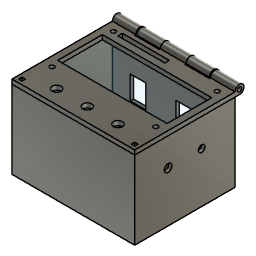
My_STM32_Box v11 (Autodesk Fusion 360 design; units mm, degrees)
Autodesk Fusion 360 part; units mm, degrees
note: some values were not read from the file. Set by a fixed rule: which sketch regions a step uses.
sketch "Sketch1" plane through (0, 0, 0) normal (0, 0, 1) x (1, 0, 0)
  line L0 (0, 0) -> (110, 0)
  line L1 (110, 0) -> (110, 70)
  line L2 (110, 70) -> (0, 70)
  line L3 (0, 70) -> (0, 0)
  dimension "d1" = 110
  dimension "d2" = 70
  constraint horizontal L0
  constraint vertical L1
  constraint horizontal L2
  constraint vertical L3
  constraint coincident L0.start L3.end
  measures "d1" distance of L0.start L0.end
  measures "d2" distance of L0.start L2.end
sketch "Sketch2" plane through (0, 0, 3) normal (0, 0, 1) x (-1, 0, 0)
  line L0 (0, -70) -> (0, 0)
  line L1 (0, 0) -> (-110, 0)
  line L2 (-110, 0) -> (-110, -70)
  line L3 (-110, -70) -> (0, -70)
  line L4 (-5, -14) -> (-105, -14)
  line L5 (-105, -14) -> (-105, -56)
  line L6 (-105, -56) -> (-5, -56)
  line L7 (-5, -56) -> (-5, -14)
  dimension "d10" = 100
  dimension "d11" = 42
  constraint horizontal L4
  constraint vertical L5
  constraint horizontal L6
  constraint vertical L7
  measures "d10" distance of L4.start L4.end
  measures "d11" distance of L4.start L6.end
sketch "Sketch3" plane through (0, 0, 3) normal (0, 0, 1) x (-1, 0, 0)
  line L0 (-105, -14) -> (-5, -14)
  line L1 (-5, -14) -> (-5, -56)
  line L2 (-5, -56) -> (-105, -56)
  line L3 (-105, -56) -> (-105, -14)
  line L4 (0, -70) -> (0, 0)
  line L5 (0, 0) -> (-110, 0)
  line L6 (-110, 0) -> (-110, -70)
  line L7 (-110, -70) -> (0, -70)
  line L8 (-12, -63) -> (-55, -63)
  line L9 (-55, -63) -> (-55, -65)
  line L10 (-55, -65) -> (-12, -65)
  line L11 (-12, -65) -> (-12, -63)
  dimension "d14" = 43
  dimension "d15" = 2
  constraint horizontal L8
  constraint vertical L9
  constraint horizontal L10
  constraint vertical L11
  measures "d14" distance of L8.start L8.end
  measures "d15" distance of L8.start L10.end
sketch "Sketch4" plane through (0, 0, 3) normal (0, 0, 1) x (-1, 0, 0)
  line L0 (-55, -63) -> (-12, -63)
  line L1 (-12, -63) -> (-12, -65)
  line L2 (-12, -65) -> (-55, -65)
  line L3 (-55, -65) -> (-55, -63)
  line L4 (-105, -14) -> (-5, -14)
  line L5 (-5, -14) -> (-5, -56)
  line L6 (-5, -56) -> (-105, -56)
  line L7 (-105, -56) -> (-105, -14)
  line L8 (0, -70) -> (0, 0)
  line L9 (0, 0) -> (-110, 0)
  line L10 (-110, 0) -> (-110, -70)
  line L11 (-110, -70) -> (0, -70)
  circle A0 centre (-7.3, -7.3) radius 2
  dimension "d18" = 4
  measures "d18" diameter of A0
sketch "Sketch5" plane through (0, 0, 3) normal (0, 0, 1) x (-1, 0, 0)
  circle A0 centre (-7.3, -7.3) radius 2
  line L0 (-55, -63) -> (-12, -63)
  line L1 (-12, -63) -> (-12, -65)
  line L2 (-12, -65) -> (-55, -65)
  line L3 (-55, -65) -> (-55, -63)
  line L4 (-105, -14) -> (-5, -14)
  line L5 (-5, -14) -> (-5, -56)
  line L6 (-5, -56) -> (-105, -56)
  line L7 (-105, -56) -> (-105, -14)
  line L8 (0, -70) -> (0, 0)
  line L9 (0, 0) -> (-110, 0)
  line L10 (-110, 0) -> (-110, -70)
  line L11 (-110, -70) -> (0, -70)
  circle A1 centre (-102.7, -7.3) radius 2
  dimension "d21" = 4
  measures "d21" diameter of A1
sketch "Sketch6" plane through (0, 0, 3) normal (0, 0, 1) x (-1, 0, 0)
sketch "Sketch7" plane through (0, 0, 0) normal (0, 0, 1) x (1, 0, 0)
  line L0 (0, 0) -> (110, 0)
  line L1 (110, 0) -> (110, 70)
  line L2 (110, 70) -> (0, 70)
  line L3 (0, 70) -> (0, 0)
  dimension "d24" = 110
  dimension "d25" = 70
  constraint horizontal L0
  constraint vertical L1
  constraint horizontal L2
  constraint vertical L3
  constraint coincident L0.start L3.end
  measures "d24" distance of L0.start L0.end
  measures "d25" distance of L0.start L2.end
extrude "Extrude7" add sketch "Sketch7" along normal blind 4 makes body 1
sketch "Sketch8" plane through (0, 0, 4) normal (0, 0, 1) x (-1, 0, 0)
  line L0 (0, -70) -> (0, 0)
  line L1 (0, 0) -> (-110, 0)
  line L2 (-110, 0) -> (-110, -70)
  line L3 (-110, -70) -> (0, -70)
  line L4 (0, 0) -> (-8.5, 0)
  line L5 (-8.5, 0) -> (-8.5, -7.5)
  line L6 (-8.5, -7.5) -> (-101.5, -7.5)
  line L7 (-101.5, -62.5) -> (-8.5, -62.5)
  circle A0 centre (-8.5, -62.5) radius 2
  circle A1 centre (-101.5, -62.5) radius 2
  circle A2 centre (-8.5, -7.5) radius 2
  circle A3 centre (-101.5, -7.5) radius 2
  line L8 (0, 0) -> (-4, 0)
  line L9 (-4, 0) -> (-4, -13)
  line L10 (-4, -13) -> (0, -13)
  line L11 (0, -13) -> (0, 0)
  line L12 (-4, -13) -> (-106, -13)
  line L13 (-106, -13) -> (-106, -57)
  line L14 (-106, -57) -> (-4, -57)
  line L15 (-4, -57) -> (-4, -13)
  line L16 (-14, -61) -> (-56, -61)
  line L17 (-56, -61) -> (-56, -65)
  line L18 (-56, -65) -> (-14, -65)
  line L19 (-14, -65) -> (-14, -61)
  dimension "d28" = 8.5
  dimension "d29" = 7.5
  dimension "d30" = 93
  dimension "d31" = 55
  dimension "d32" = 4
  dimension "d33" = 4
  dimension "d34" = 4
  dimension "d35" = 4
  dimension "d36" = 4
  dimension "d37" = 13
  dimension "d38" = 102
  dimension "d39" = 44
  dimension "d40" = 42
  constraint coincident L0.end L1.start
  constraint perpendicular L0 L4
  constraint perpendicular L4 L5
  constraint horizontal L6
  constraint horizontal L7
  constraint coincident L7.end A0.centre
  constraint coincident L7.start A1.centre
  constraint coincident L5.end L6.start
  constraint coincident L6.end A3.centre
  constraint horizontal L8
  constraint vertical L9
  constraint horizontal L10
  constraint vertical L11
  constraint horizontal L12
  constraint vertical L13
  constraint horizontal L14
  constraint vertical L15
  constraint horizontal L16
  constraint vertical L17
  constraint horizontal L18
  constraint vertical L19
  measures "d28" distance of L0.end L4.end
  measures "d29" distance of L4.end L5.end
  measures "d30" distance of L5.end L6.end
  measures "d31" distance of L5.end L7.end
  measures "d32" diameter of A0
  measures "d33" diameter of A1
  measures "d34" diameter of A2
  measures "d35" diameter of A3
  measures "d36" distance of L0.end L8.end
  measures "d37" distance of L0.end L10.end
  measures "d38" distance of L9.end L12.end
  measures "d39" distance of L9.end L14.end
  measures "d40" distance of L16.start L16.end
extrude "Extrude8" cut sketch "Sketch8" against normal blind 4 contours L12 L13 L14 L15 | L5 L6 A2 | L5 L6 A2 | L7 L16 L17 L19 | L7 L17 L18 L19 | A0 | A1 | A3 bodies 1
sketch "Sketch9" plane through (110, 0, 0) normal (1, 0, 0) x (0, 1, 0)
  line L0 (0, 0) -> (70, 0)
  line L1 (70, 0) -> (70, 4)
  line L2 (70, 4) -> (0, 4)
  line L3 (0, 4) -> (0, 0)
sketch "Sketch10" plane through (110, 0, 0) normal (1, 0, 0) x (0, 1, 0)
sketch "Sketch11" plane through (0, 0, 0) normal (-1, 0, 0) x (0, -1, 0)
  line L0 (-70, 0) -> (0, 0)
  line L1 (0, 0) -> (0, 4)
  line L2 (0, 4) -> (-70, 4)
  line L3 (-70, 4) -> (-70, 0)
sketch "Sketch12" plane through (0, 0, 4) normal (0, 0, 1) x (-1, 0, 0)
  line L0 (-106, -13) -> (-4, -13)
  line L1 (-4, -13) -> (-4, -57)
  line L2 (-4, -57) -> (-106, -57)
  line L3 (-106, -57) -> (-106, -13)
  circle A0 centre (-8.5, -62.5) radius 2
  circle A1 centre (-101.5, -7.5) radius 2
  circle A2 centre (-8.5, -7.5) radius 2
  line L4 (-56, -61) -> (-14, -61)
  line L5 (-14, -61) -> (-14, -65)
  line L6 (-14, -65) -> (-56, -65)
  line L7 (-56, -65) -> (-56, -61)
  circle A3 centre (-101.5, -62.5) radius 2
  line L8 (0, -70) -> (0, 0)
  line L9 (0, 0) -> (-110, 0)
  line L10 (-110, 0) -> (-110, -70)
  line L11 (-110, -70) -> (0, -70)
  line L12 (0, -70) -> (-44, -70)
  line L13 (0, -70) -> (-65, -70)
  line L14 (0, -70) -> (-88, -70)
  dimension "d43" = 44
  dimension "d44" = 65
  dimension "d45" = 88
  constraint coincident L8.start L11.end
  constraint perpendicular L8 L12
  constraint perpendicular L8 L13
  constraint parallel L11 L14
  measures "d43" distance of L8.start L12.end
  measures "d44" distance of L8.start L13.end
  measures "d45" distance of L8.start L14.end
sketch "Sketch13" plane through (0, 0, 4) normal (0, 0, 1) x (-1, 0, 0)
  line L0 (0, -70) -> (-21, -70)
  dimension "d46" = 21
  constraint horizontal L0
  measures "d46" distance of L0.start L0.end
sketch "Sketch14" plane through (110, 0, 0) normal (1, 0, 0) x (0, 1, 0)
  circle A0 centre (74, 4) radius 4
  line L0 (74, 0) -> (70, 0)
  line L1 (70, 0) -> (70, 4)
  circle A1 centre (74, 4) radius 2
  dimension "d47" = 4
  constraint coincident A0 L0.start
  constraint tangent A0 L0
  constraint horizontal L0
  constraint coincident A0 L1.end
  constraint tangent A0 L1
  constraint perpendicular L0 L1
  constraint concentric A0 A1
  measures "d47" diameter of A1
sketch "Sketch15" plane through (0, 70, 0) normal (0, 1, 0) x (-1, 0, 0)
  line L0 (-110, 0) -> (0, 0)
  line L1 (0, 0) -> (0, 4)
  line L2 (0, 4) -> (-110, 4)
  line L3 (-110, 4) -> (-110, 0)
sketch "Sketch16" plane through (0, 0, 0) normal (-1, 0, 0) x (0, -1, 0)
  circle A0 centre (74, 4) radius 2
  circle A1 centre (74, 4) radius 4
  circle A2 centre (-74, 4) radius 4
  circle A3 centre (-74, 4) radius 2
  line L0 (-74, 0) -> (-70, 0)
  line L1 (-70, 0) -> (-70, 4)
  dimension "d48" = 4
  constraint concentric A0 A1
  constraint concentric A2 A3
  constraint coincident A2 L0.start
  constraint tangent A2 L0
  constraint horizontal L0
  constraint coincident A2 L1.end
  constraint tangent A2 L1
  constraint perpendicular L0 L1
  measures "d48" diameter of A0
extrude "Extrude9" add sketch "Sketch14" against normal blind 22 bodies 1
extrude "Extrude10" add sketch "Sketch16" against normal blind 21 contours A2 | A2 L0 L1 bodies 1
extrude "Extrude11" add 1 faces at (21, 72.3333, 0.756) along direction (1, 0, 0) blind 45 on bodies 1 bodies 1
sketch "Sketch17" plane through (66, 0, 0) normal (1, 0, 0) x (0, 1, 0)
  circle A0 centre (74, 4) radius 2
  line L0 (70, 4) -> (70, 0)
  line L1 (70, 0) -> (74, 0)
  arc A1 (74, 0) -> (70, 4) centre (74, 4) ccw
  circle A2 centre (74, 4) radius 4
  circle A3 centre (74, 4) radius 2
  constraint concentric A0 A2
  constraint coincident L0.start A2
  constraint concentric A2 A3
sketch "Sketch18" plane through (0, 0, 4) normal (0, 0, 1) x (-1, 0, 0)
  line L0 (-44, -70) -> (-21, -70)
  line L1 (-21, -70) -> (-21, -78.7723)
  line L2 (-44, -78.7723) -> (-44, -70)
  constraint horizontal L0
  constraint vertical L1
  constraint vertical L2
sketch "Sketch19" plane through (0, 0, 4) normal (0, 0, 1) x (1, 0, 0)
sketch "Sketch20" plane through (0, 0, 0) normal (1, 0, 0) x (0, 1, 0)
  circle A0 centre (74, 4) radius 2
  circle A1 centre (74, 4) radius 4
  constraint concentric A0 A1
sketch "Sketch21" plane through (0, 0, 0) normal (-1, 0, 0) x (0, -1, 0)
sketch "Sketch22" plane through (0, 70, 0) normal (0, 1, 0) x (-1, 0, 0)
  line L0 (-43, 0) -> (-21, 0)
  line L1 (-21, 0) -> (-21, 8)
  line L2 (-21, 8) -> (-43, 8)
  line L3 (-43, 8) -> (-43, 0)
  constraint horizontal L0
  constraint vertical L1
  constraint horizontal L2
  constraint vertical L3
extrude "Extrude12" cut sketch "Sketch22" along normal blind 8 bodies 1
move_body "Move1" bodies 1 to x (1, 0, 0) y (0, 1, 0) z (0, 0, 1) at (0, 0, 60)
move_body "Move2" bodies 1 to x (1, 0, 0) y (0, 1, 0) z (0, 0, 1) at (0, 100, 0)
sketch "Sketch23" plane through (0, 0, 0) normal (0, 0, 1) x (1, 0, 0)
extrude "Extrude13" add 1 faces at (36.6667, 100, 61.3333) along direction (0, -1, 0) blind 20 on bodies 1 bodies 1
sketch "Sketch24" plane through (0, 0, 64) normal (0, 0, 1) x (-1, 0, 0)
  line L0 (-106, -113) -> (-4, -113)
  line L1 (-4, -113) -> (-4, -157)
  line L2 (-4, -157) -> (-106, -157)
  line L3 (-106, -157) -> (-106, -113)
  circle A0 centre (-8.5, -162.5) radius 2
  circle A1 centre (-101.5, -107.5) radius 2
  circle A2 centre (-8.5, -107.5) radius 2
  line L4 (-56, -161) -> (-14, -161)
  line L5 (-14, -161) -> (-14, -165)
  line L6 (-14, -165) -> (-56, -165)
  line L7 (-56, -165) -> (-56, -161)
  circle A3 centre (-101.5, -162.5) radius 2
  line L8 (0, -170) -> (0, -80)
  line L9 (0, -80) -> (-110, -80)
  line L10 (-110, -80) -> (-110, -170)
  line L11 (-110, -170) -> (-88, -170)
  line L12 (-88, -170) -> (-66, -170)
  line L13 (-66, -170) -> (-43, -170)
  line L14 (-43, -170) -> (-21, -170)
  line L15 (-21, -170) -> (0, -170)
  line L16 (0, -80) -> (-27.5, -80)
  line L17 (0, -80) -> (-55, -80)
  line L18 (-55, -80) -> (-82.5, -80)
  line L19 (-27.5, -80) -> (-27.5, -92.5)
  line L20 (-27.5, -92.5) -> (-55, -92.5)
  line L21 (-55, -92.5) -> (-82.5, -92.5)
  circle A4 centre (-27.5, -92.5) radius 4
  circle A5 centre (-55, -92.5) radius 4
  circle A6 centre (-82.5, -92.5) radius 4
  dimension "d62" = 27.5
  dimension "d63" = 27.5
  dimension "d64" = 12.5
  dimension "d65" = 27.5
  dimension "d66" = 8
  dimension "d67" = 8
  dimension "d68" = 8
  constraint coincident L8.end L9.start
  constraint perpendicular L8 L16
  constraint midpoint L9 L17.end
  constraint parallel L9 L18
  constraint perpendicular L16 L19
  constraint perpendicular L19 L20
  constraint parallel L18 L21
  constraint coincident L19.end L20.start
  constraint coincident L20.end L21.start
  constraint coincident L21.end A6.centre
  measures "d62" distance of L8.end L16.end
  measures "d63" distance of L17.end L18.end
  measures "d64" distance of L16.end L19.end
  measures "d65" distance of L20.end L21.end
  measures "d66" diameter of A4
  measures "d67" diameter of A5
  measures "d68" diameter of A6
extrude "Extrude14" cut sketch "Sketch24" against normal blind 4 contours L19 L20 A4 | L19 L20 A4 | L20 L21 A5 | L20 L21 A5 | A6 bodies 1
sketch "Sketch25" plane through (0, 0, 0) normal (0, 0, 1) x (1, 0, 0)
  line L0 (0, 0) -> (110, 0)
  line L1 (110, 0) -> (110, 90)
  line L2 (110, 90) -> (0, 90)
  line L3 (0, 90) -> (0, 0)
  dimension "d71" = 110
  dimension "d72" = 90
  constraint horizontal L0
  constraint vertical L1
  constraint horizontal L2
  constraint vertical L3
  constraint coincident L0.start L3.end
  measures "d71" distance of L0.start L0.end
  measures "d72" distance of L0.start L2.end
move_body "Move3" bodies 1 to x (1, 0, 0) y (0, 1, 0) z (0, 0, 1) at (0, -80, 0)
move_body "Move4" bodies 1 to x (1, 0, 0) y (0, 1, 0) z (0, 0, 1) at (0, 100, 0)
sketch "Sketch26" plane through (0, 0, 0) normal (0, 0, 1) x (1, 0, 0)
  line L0 (0, 90) -> (9, 90)
  line L1 (9, 90) -> (9, 85)
  line L2 (9, 85) -> (0, 85)
  line L3 (0, 85) -> (0, 90)
  line L4 (9, 85) -> (13.45, 85)
  line L5 (13.45, 85) -> (13.45, 80.55)
  line L6 (13.45, 80.55) -> (9, 80.55)
  line L7 (9, 80.55) -> (9, 85)
  line L8 (13.45, 80.55) -> (96, 80.55)
  line L9 (96, 80.55) -> (96, 24.7)
  line L10 (96, 24.7) -> (13.45, 24.7)
  line L11 (13.45, 24.7) -> (13.45, 80.55)
  circle A0 centre (13.45, 24.7) radius 2
  circle A1 centre (13.45, 80.55) radius 2
  circle A2 centre (96, 80.55) radius 2
  circle A3 centre (96, 24.7) radius 2
  line L12 (3, 87) -> (107, 87)
  line L13 (107, 87) -> (107, 3)
  line L14 (107, 3) -> (3, 3)
  line L15 (3, 3) -> (3, 87)
  line L16 (9, 85) -> (100.5298, 85)
  line L17 (100.5298, 85) -> (100.5298, 20.5176)
  line L18 (100.5298, 20.5176) -> (9, 20.5176)
  line L19 (9, 20.5176) -> (9, 85)
  dimension "d73" = 9
  dimension "d74" = 5
  dimension "d75" = 4.45
  dimension "d76" = 4.45
  dimension "d77" = 82.55
  dimension "d78" = 55.85
  dimension "d79" = 4
  dimension "d80" = 4
  dimension "d81" = 4
  dimension "d82" = 4
  constraint horizontal L0
  constraint vertical L1
  constraint horizontal L2
  constraint vertical L3
  constraint horizontal L4
  constraint vertical L5
  constraint horizontal L6
  constraint vertical L7
  constraint horizontal L8
  constraint vertical L9
  constraint horizontal L10
  constraint vertical L11
  constraint coincident L10.end L11.start
  constraint coincident L5.end L6.start
  constraint coincident L8.end L9.start
  constraint coincident L9.end L10.start
  constraint horizontal L12
  constraint vertical L13
  constraint horizontal L14
  constraint vertical L15
  constraint horizontal L16
  constraint vertical L17
  constraint horizontal L18
  constraint vertical L19
  measures "d73" distance of L0.start L0.end
  measures "d74" distance of L0.start L2.end
  measures "d75" distance of L1.end L4.end
  measures "d76" distance of L1.end L6.end
  measures "d77" distance of L5.end L8.end
  measures "d78" distance of L5.end L10.end
  measures "d79" diameter of A0
  measures "d80" diameter of A1
  measures "d81" diameter of A2
  measures "d82" diameter of A3
extrude "Extrude15" add sketch "Sketch25" sketch "Sketch26" along normal blind 70 separate body of sketch 2 contours L1 L2 L12 L13 L14 L15 makes body 2
sketch "Sketch27" plane through (0, 0, 70) normal (0, 0, 1) x (-1, 0, 0)
  line L0 (0, -90) -> (0, 0)
  line L1 (0, 0) -> (-110, 0)
  line L2 (-110, 0) -> (-110, -90)
  line L3 (-110, -90) -> (0, -90)
  line L4 (-3, -3) -> (-107, -3)
  line L5 (-107, -3) -> (-107, -87)
  line L6 (-107, -87) -> (-3, -87)
  line L7 (-3, -87) -> (-3, -3)
  constraint horizontal L4
  constraint vertical L5
  constraint horizontal L6
  constraint vertical L7
extrude "Extrude16" cut sketch "Sketch27" against normal blind 67 contours L4 L5 L6 L7 bodies 2
sketch "Sketch28" plane through (0, 0, 3) normal (0, 0, 1) x (-1, 0, 0)
  line L0 (-3, -87) -> (-3, -3)
  line L1 (-3, -3) -> (-107, -3)
  line L2 (-107, -3) -> (-107, -87)
  line L3 (-107, -87) -> (-3, -87)
  line L4 (0, -90) -> (-9, -90)
  line L5 (-9, -90) -> (-9, -85)
  line L6 (-9, -85) -> (0, -85)
  line L7 (0, -85) -> (0, -90)
  line L8 (-9, -85) -> (-13.45, -85)
  line L9 (-13.45, -85) -> (-13.45, -80.55)
  line L10 (-13.45, -80.55) -> (-9, -80.55)
  line L11 (-9, -80.55) -> (-9, -85)
  line L12 (-13.45, -80.55) -> (-95.95, -80.55)
  line L13 (-95.95, -80.55) -> (-95.95, -24.75)
  line L14 (-95.95, -24.75) -> (-13.45, -24.75)
  line L15 (-13.45, -24.75) -> (-13.45, -80.55)
  circle A0 centre (-13.45, -80.55) radius 2
  circle A1 centre (-95.95, -80.55) radius 2
  circle A2 centre (-95.95, -24.75) radius 2
  circle A3 centre (-13.45, -24.75) radius 2
  dimension "d87" = 4.45
  dimension "d88" = 4.45
  dimension "d89" = 82.5
  dimension "d90" = 55.8
  dimension "d91" = 4
  dimension "d92" = 4
  dimension "d93" = 4
  dimension "d94" = 4
  constraint horizontal L4
  constraint vertical L5
  constraint horizontal L6
  constraint vertical L7
  constraint horizontal L8
  constraint vertical L9
  constraint horizontal L10
  constraint vertical L11
  constraint horizontal L12
  constraint vertical L13
  constraint horizontal L14
  constraint vertical L15
  constraint coincident L9.end L10.start
  constraint coincident L12.end L13.start
  constraint coincident L13.end L14.start
  constraint coincident L14.end L15.start
  measures "d87" distance of L5.end L8.end
  measures "d88" distance of L5.end L10.end
  measures "d89" distance of L9.end L12.end
  measures "d90" distance of L9.end L14.end
  measures "d91" diameter of A0
  measures "d92" diameter of A1
  measures "d93" diameter of A2
  measures "d94" diameter of A3
extrude "Extrude17" cut sketch "Sketch28" against normal blind 3 contours L9 L12 A0 | L9 L10 A0 | L10 L15 A0 | L12 L15 A0 | L12 L13 A1 | L12 L13 A1 | L14 L15 A3 | L14 L15 A3 | L13 L14 A2 | L13 L14 A2 bodies 2
sketch "Sketch29" plane through (0, 87, 0) normal (0, -1, 0) x (1, 0, 0)
  line L0 (107, 70) -> (3, 70)
  line L1 (3, 70) -> (3, 3)
  line L2 (3, 3) -> (107, 3)
  line L3 (107, 3) -> (107, 70)
sketch "Sketch30" plane through (0, 87, 0) normal (0, -1, 0) x (1, 0, 0)
  line L0 (32, 70) -> (20, 70)
  line L1 (0, 23) -> (60, 23)
  line L2 (60, 23) -> (75, 23)
  line L3 (60, 23) -> (75, 23)
  line L4 (75, 23) -> (75, 70)
  line L5 (75, 70) -> (60, 70)
  line L6 (60, 70) -> (60, 23)
  line L7 (19, 23) -> (33, 23)
  line L8 (33, 23) -> (33, 70)
  line L9 (33, 70) -> (19, 70)
  line L10 (19, 70) -> (19, 23)
  constraint horizontal L0
  constraint horizontal L1
  constraint parallel L1 L2
  constraint horizontal L3
  constraint vertical L4
  constraint horizontal L5
  constraint vertical L6
  constraint horizontal L7
  constraint vertical L8
  constraint horizontal L9
  constraint vertical L10
  constraint coincident L1 L7.start
extrude "Extrude18" cut sketch "Sketch30" against normal blind 3 bodies 2
sketch "Sketch31" plane through (19, 0, 0) normal (1, 0, 0) x (0, 1, 0)
  line L0 (87, 70) -> (87, 23)
  line L1 (87, 23) -> (90, 23)
  line L2 (90, 23) -> (90, 70)
  line L3 (90, 70) -> (87, 70)
  line L4 (90, 70) -> (87, 70)
  line L5 (87, 70) -> (87, 64)
  line L6 (87, 64) -> (90, 64)
  line L7 (90, 64) -> (90, 70)
  constraint horizontal L4
  constraint vertical L5
  constraint horizontal L6
  constraint vertical L7
  constraint coincident L0 L5.end
  constraint coincident L2.end L3.start
extrude "Extrude19" add sketch "Sketch31" along normal blind 56 contours L0 L2 L3 L4 L5 L6 L7 bodies 2
extrude "Extrude20" add 2 faces at (65, 88, 64) (23.6667, 88, 64) along direction (0, 0, -1) blind 5 on bodies 2 bodies 2
sketch "Sketch32" plane through (3, 0, 0) normal (1, 0, 0) x (0, 1, 0)
  line L0 (87, 70) -> (3, 70)
  line L1 (3, 70) -> (3, 3)
  line L2 (3, 3) -> (87, 3)
  line L3 (87, 3) -> (87, 70)
sketch "Sketch33" plane through (3, 0, 0) normal (1, 0, 0) x (0, 1, 0)
  line L0 (90, 0) -> (51, 0)
  line L1 (51, 0) -> (51, 20)
  line L2 (51, 20) -> (90, 20)
  line L3 (90, 20) -> (90, 0)
  line L4 (51, 20) -> (39, 20)
  line L5 (39, 20) -> (39, 32)
  line L6 (39, 32) -> (51, 32)
  line L7 (51, 32) -> (51, 20)
  dimension "d105" = 39
  dimension "d106" = 20
  dimension "d107" = 12
  dimension "d108" = 12
  constraint horizontal L0
  constraint vertical L1
  constraint horizontal L2
  constraint vertical L3
  constraint horizontal L4
  constraint vertical L5
  constraint horizontal L6
  constraint vertical L7
  measures "d105" distance of L0.start L0.end
  measures "d106" distance of L0.start L2.end
  measures "d107" distance of L1.end L4.end
  measures "d108" distance of L1.end L6.end
extrude "Extrude21" cut sketch "Sketch33" against normal blind 3 contours L4 L5 L6 L7 bodies 2
move_body "Move5" bodies 1 to x (1, 0, 0) y (0, 1, 0) z (0, 0, 1) at (0, -100, 10)
move_body "Move6" bodies 1 to x (1, 0, 0) y (0, 1, 0) z (0, 0, 1) at (0, 115, 0)
sketch "Sketch34" plane through (110, 0, 0) normal (1, 0, 0) x (0, 1, 0)
  line L0 (0, 0) -> (90, 0)
  line L1 (90, 0) -> (90, 70)
  line L2 (90, 70) -> (0, 70)
  line L3 (0, 70) -> (0, 0)
  line L4 (90, 70) -> (94, 70)
  line L5 (94, 70) -> (94, 74)
  circle A0 centre (94, 74) radius 4
  circle A1 centre (94, 74) radius 2
  line L6 (90, 70) -> (90, 74)
  line L7 (97.4213, 71.9275) -> (90, 59.0464)
  constraint coincident L1.end L2.start
  constraint perpendicular L1 L4
  constraint perpendicular L4 L5
  constraint coincident L5.end A0.centre
  constraint coincident L4.end A0
  constraint concentric A0 A1
  constraint coincident A0 L6.end
  constraint tangent A0 L6
  constraint coincident A0 L7.start
  constraint coincident L1 L7.end
extrude "Extrude22" add sketch "Sketch34" against normal blind 110 contours L1 L4 A0 L7 | L4 A0 L6 | A0 bodies 2
sketch "Sketch35" plane through (0, 90, 0) normal (0, 1, 0) x (-1, 0, 0)
  line L0 (0, 59.0464) -> (-110, 59.0464)
  line L1 (-110, 59.0464) -> (-110, 0)
  line L2 (-110, 0) -> (0, 0)
  line L3 (0, 0) -> (0, 59.0464)
  line L4 (-19, 59) -> (-19, 23)
  line L5 (-19, 23) -> (-33, 23)
  line L6 (-33, 23) -> (-33, 59)
  line L7 (-33, 59) -> (-19, 59)
  line L8 (-60, 59) -> (-60, 23)
  line L9 (-60, 23) -> (-75, 23)
  line L10 (-75, 23) -> (-75, 59)
  line L11 (-75, 59) -> (-60, 59)
  line L12 (0, 59.0464) -> (-22, 59.0464)
  line L13 (0, 59.0464) -> (-43, 59.0464)
  line L14 (0, 59.0464) -> (-66, 59.0464)
  line L15 (0, 59.0464) -> (-87, 59.0464)
  line L16 (-22, 59.0464) -> (0, 59.0464)
  line L17 (0, 59.0464) -> (0, 80)
  line L18 (0, 80) -> (-22, 80)
  line L19 (-22, 80) -> (-22, 59.0464)
  line L20 (-43, 59.0464) -> (-66, 59.0464)
  line L21 (-66, 59.0464) -> (-66, 79)
  line L22 (-66, 79) -> (-43, 79)
  line L23 (-43, 79) -> (-43, 59.0464)
  line L24 (-87, 59.0464) -> (-110, 59.0464)
  line L25 (-110, 59.0464) -> (-110, 82)
  line L26 (-110, 82) -> (-87, 82)
  line L27 (-87, 82) -> (-87, 59.0464)
  dimension "d113" = 22
  dimension "d114" = 43
  dimension "d115" = 66
  dimension "d116" = 87
  constraint coincident L0.start L3.end
  constraint perpendicular L3 L12
  constraint horizontal L13
  constraint perpendicular L8 L14
  constraint parallel L0 L15
  constraint horizontal L16
  constraint vertical L17
  constraint horizontal L18
  constraint vertical L19
  constraint horizontal L20
  constraint vertical L21
  constraint horizontal L22
  constraint vertical L23
  constraint horizontal L24
  constraint vertical L25
  constraint horizontal L26
  constraint vertical L27
  measures "d113" distance of L0.start L12.end
  measures "d114" distance of L0.start L13.end
  measures "d115" distance of L0.start L14.end
  measures "d116" distance of L0.start L15.end
extrude "Extrude23" cut sketch "Sketch35" along normal blind 10 contours L0 L12 L13 L14 L15 L16 L17 L18 L19 | L0 L14 L15 L20 L21 L22 L23 | L0 L24 L25 L26 L27 bodies 2
move_body "Move7" bodies 1 to x (1, 0, 0) y (0, 1, 0) z (0, 0, 1) at (0, -115, 0)
extrude "Extrude24" cut 1 faces at (2, 39, 24) along direction (0, -1, 0) blind 3 on bodies 2 bodies 2
sketch "Sketch36" plane through (87, 0, 0) normal (1, 0, 0) x (0, 1, 0)
  line L0 (90, 59.0464) -> (97.4213, 71.9275)
  arc A0 (97.4213, 71.9275) -> (90, 74) centre (94, 74) ccw
  line L1 (90, 74) -> (90, 70)
  line L2 (90, 70) -> (90, 59.0464)
  circle A1 centre (94, 74) radius 2
  line L3 (90, 70) -> (98, 70)
  line L4 (98, 70) -> (98, 0)
  line L5 (98, 0) -> (90, 0)
  line L6 (90, 0) -> (90, 70)
  line L7 (98, 70) -> (98, 74)
  dimension "d121" = 8
  dimension "d122" = 70
  constraint horizontal L3
  constraint vertical L4
  constraint horizontal L5
  constraint vertical L6
  constraint coincident L1.end L2.start
  constraint coincident A0 L7.end
  constraint tangent A0 L7
  measures "d121" distance of L1.end L3.end
  measures "d122" distance of L1.end L5.end
extrude "Extrude25" add sketch "Sketch36" against normal blind 12 contours L0 L3 L4 L5 L6 | L0 A0 L3 L7 bodies 2
sketch "Sketch37" plane through (22, 0, 0) normal (-1, 0, 0) x (0, -1, 0)
  line L0 (-97.4213, 71.9275) -> (-90, 59.0464)
  line L1 (-90, 59.0464) -> (-90, 70)
  line L2 (-90, 70) -> (-90, 74)
  arc A0 (-90, 74) -> (-97.4213, 71.9275) centre (-94, 74) ccw
  circle A1 centre (-94, 74) radius 2
sketch "Sketch38" plane through (43, 0, 0) normal (1, 0, 0) x (0, 1, 0)
  line L0 (90, 59.0464) -> (97.4213, 71.9275)
  arc A0 (97.4213, 71.9275) -> (90, 74) centre (94, 74) ccw
  line L1 (90, 74) -> (90, 70)
  line L2 (90, 70) -> (90, 59.0464)
  circle A1 centre (94, 74) radius 2
  line L3 (90, 70) -> (98, 70)
  line L4 (98, 70) -> (98, 0)
  line L5 (98, 0) -> (90, 0)
  line L6 (90, 0) -> (90, 70)
  line L7 (98, 70) -> (98, 74)
  dimension "d125" = 8
  dimension "d126" = 70
  constraint horizontal L3
  constraint vertical L4
  constraint horizontal L5
  constraint vertical L6
  constraint coincident L1.end L2.start
  constraint coincident A0 L7.end
  constraint tangent A0 L7
  measures "d125" distance of L1.end L3.end
  measures "d126" distance of L1.end L5.end
extrude "Extrude26" add sketch "Sketch38" against normal blind 10 contours L0 L3 L4 L5 L6 | L0 A0 L3 L7 bodies 2
move_face "OffsetFaces1" offset 2 1 faces at (4, 62.3333, 72.6667) on bodies 1
move_face "OffsetFaces2" offset 2 1 faces at (106, 47.6667, 72.6667) on bodies 1
move_face "OffsetFaces3" offset 2 1 faces at (71.3333, 77, 72.6667) on bodies 1
move_face "OffsetFaces4" offset 2 1 faces at (38.6667, 33, 72.6667) on bodies 1
move_face "OffsetFaces5" offset -1 1 faces at (80.6667, 90, 71.3333) on bodies 1
move_face "OffsetFaces6" offset -1 1 faces at (28.3333, 90, 71.3333) on bodies 1
sketch "Sketch39" plane through (0, 0, 74) normal (0, 0, 1) x (-1, 0, 0)
  circle A0 centre (-27.5, -12.5) radius 4
  circle A1 centre (-55, -12.5) radius 4
  circle A2 centre (-82.5, -12.5) radius 4
  line L0 (-104, -35) -> (-6, -35)
  line L1 (-6, -35) -> (-6, -75)
  line L2 (-6, -75) -> (-104, -75)
  line L3 (-104, -75) -> (-104, -35)
  circle A3 centre (-8.5, -82.5) radius 2
  circle A4 centre (-101.5, -27.5) radius 2
  circle A5 centre (-8.5, -27.5) radius 2
  line L4 (-56, -81) -> (-14, -81)
  line L5 (-14, -81) -> (-14, -85)
  line L6 (-14, -85) -> (-56, -85)
  line L7 (-56, -85) -> (-56, -81)
  circle A6 centre (-101.5, -82.5) radius 2
  line L8 (0, -90) -> (0, 0)
  line L9 (0, 0) -> (-110, 0)
  line L10 (-110, 0) -> (-110, -90)
  line L11 (-110, -90) -> (-88, -90)
  line L12 (-88, -90) -> (-88, -89)
  line L13 (-88, -89) -> (-66, -89)
  line L14 (-66, -89) -> (-66, -90)
  line L15 (-66, -90) -> (-43, -90)
  line L16 (-43, -90) -> (-43, -89)
  line L17 (-43, -89) -> (-21, -89)
  line L18 (-21, -89) -> (-21, -90)
  line L19 (-21, -90) -> (0, -90)
  line L20 (0, 0) -> (-3, 0)
  line L21 (-3, 0) -> (-3, -3)
  line L22 (-3, -3) -> (0, -3)
  line L23 (0, -3) -> (0, 0)
  line L24 (-3, -3) -> (-6, -3)
  line L25 (-6, -3) -> (-6, -6)
  line L26 (-6, -6) -> (-3, -6)
  line L27 (-3, -6) -> (-3, -3)
  line L28 (-110, 0) -> (-107, 0)
  line L29 (-107, 0) -> (-107, -3)
  line L30 (-107, -3) -> (-110, -3)
  line L31 (-110, -3) -> (-110, 0)
  line L32 (-107, -3) -> (-104, -3)
  line L33 (-104, -3) -> (-104, -6)
  line L34 (-104, -6) -> (-107, -6)
  line L35 (-107, -6) -> (-107, -3)
  dimension "d135" = 3
  dimension "d136" = 3
  dimension "d137" = 3
  dimension "d138" = 3
  dimension "d139" = 3
  dimension "d140" = 3
  constraint horizontal L20
  constraint vertical L21
  constraint horizontal L22
  constraint vertical L23
  constraint coincident L8.end L9.start
  constraint horizontal L24
  constraint vertical L25
  constraint horizontal L26
  constraint vertical L27
  constraint horizontal L28
  constraint vertical L29
  constraint horizontal L30
  constraint vertical L31
  constraint coincident L9.end L10.start
  constraint horizontal L32
  constraint vertical L33
  constraint horizontal L34
  constraint vertical L35
  measures "d135" distance of L8.end L20.end
  measures "d136" distance of L8.end L22.end
  measures "d137" distance of L21.end L24.end
  measures "d138" distance of L21.end L26.end
  measures "d139" distance of L29.end L32.end
  measures "d140" distance of L29.end L34.end
extrude "Extrude27" cut sketch "Sketch39" against normal blind 4 contours L24 L25 L26 L27 | L32 L33 L34 L35 bodies 1
sketch "Sketch40" plane through (110, 0, 0) normal (1, 0, 0) x (0, 1, 0)
  line L0 (90, 0) -> (90, 70)
  line L1 (90, 70) -> (0, 70)
  line L2 (0, 70) -> (0, 0)
  line L3 (0, 0) -> (90, 0)
  circle A0 centre (30, 45) radius 3.5
  circle A1 centre (60, 45) radius 3
  dimension "d143" = 7
  dimension "d144" = 6
  measures "d143" diameter of A0
  measures "d144" diameter of A1
extrude "Extrude28" cut sketch "Sketch40" against normal blind 3 contours A0 | A1 bodies 2
extrude "Extrude29" add 2 faces at (23.6667, 88, 59) (65, 88, 59) along direction (0, 0, -1) blind 15 on bodies 2 bodies 2
named bodies: "Lid", "Box"
